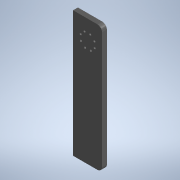
# Autodesk Inventor part: Triangle axle slide connector
Saved by Autodesk Inventor 2021 (Build 250183000, 183)
## iProperties
Part Number: Triangle axle slide connector
Material: Generic
Document SubType Name: Modeling
Designer: Delta
Appearance: Default
Author: Delta
Autodesk Inventor part; units mm, degrees
ref_plane "YZ Plane" through (0, 0, 0) normal (1, 0, 0) x (0, 1, 0)
ref_plane "XZ Plane" through (0, 0, 0) normal (0, 1, 0) x (-1, 0, 0)
ref_plane "XY Plane" through (0, 0, 0) normal (0, 0, 1) x (1, 0, 0)
sketch "Sketch1" plane through (0, 0, 0) normal (0, 0, 1) x (1, 0, 0)
  line L0 (0, 0) -> (0, 165.1)
  line L1 (0, 0) -> (53.8815, 0) construction
  line L2 (0, 165.1) -> (76.2, 165.1) construction
  line L3 (0, 165.1) -> (-38.1, 165.1)
  line L4 (-38.1, 165.1) -> (-38.1, 0)
  line L5 (0, 0) -> (-38.1, 0)
  dimension "d0" = 165.1
  dimension "d86" = 38.1
  constraints: 12 end point, 4 horizontal, 1 perpendicular, 1 vertical
  measures "d0" distance of L0.start L0.end
  measures "d86" distance of L0.end L3.end
extrude "Extrusion1" add sketch "Sketch1" along normal blind 6.35
fillet "Fillet1" radius 6.35 2 edges at (0, 165.1, 3.175) (0, 0, 3.175)
sketch "Sketch8" plane through (0, 0, 0) normal (0, 0, -1) x (-1, 0, 0)
  circle A0 centre (18.9128, 139.7) radius 2.54
  circle A1 centre (10.0465, 143.8252) radius 1.3589
  circle A2 centre (9.7264, 136.3476) radius 1.3589
  circle A3 centre (14.7876, 130.8337) radius 1.3589
  circle A4 centre (22.2652, 130.5136) radius 1.3589
  circle A5 centre (27.7791, 135.5748) radius 1.3589
  circle A6 centre (28.0992, 143.0524) radius 1.3589
  circle A7 centre (23.038, 148.5663) radius 1.3589
  circle A8 centre (15.5603, 148.8864) radius 1.3589
  line L0 (38.1, 0) -> (6.35, 0) projected
  point P0 (0, 0)
  dimension "d60" = 5.08
  dimension "d61" = 2.7178
  dimension "d62" = 9.779
  dimension "d65" = 360
  dimension "d87" = 139.7
  constraints: 9 centre point, 17 other
  measures "d60" diameter of A0
  measures "d61" diameter of A1
  measures "d62" distance of A1.centre A0.centre
  measures "d87" distance from line of A0.centre L0
extrude "Extrusion7" cut sketch "Sketch8" against normal blind 25.4 contours A1 | A2 | A3 | A4 | A5 | A6 | A7 | A8
sketch "Sketch9" plane through (0, 0, 6.35) normal (0, 0, 1) x (1, 0, 0)
  circle A0 centre (-23.038, 148.5663) radius 1.3589 projected
  circle A1 centre (-14.7876, 130.8337) radius 1.3589 projected
  circle A2 centre (-27.7791, 135.5748) radius 1.3589 projected
  point P0 (0, 0)
  point P1 (-23.2077, 143.9949)
  dimension "d69" = 16.8402
  dimension "d70" = 8.4201
  dimension "d71" = 8.4201
  measures "d70" horizontal distance of A1.centre point (-23.208, 143.995)
  measures "d71" vertical distance of point (-23.208, 143.995) A2.centre
equation "\"d70\" = 0.5 * d69"
equation "\"d71\" = d70"
body "Solid1"
